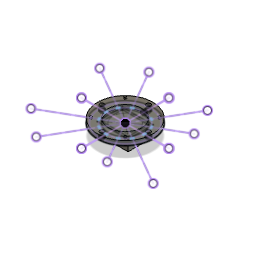
bottom_frame v1 (Autodesk Fusion 360 design; units mm, degrees)
Autodesk Fusion 360 part; units mm, degrees
note: some values were not read from the file. Set by a fixed rule: which sketch regions a step uses.
sketch "스케치1" plane through (0, 0, 0) normal (0, 1, 0) x (1, 0, 0)
  circle A0 centre (0, 0) radius 28 construction
  circle A1 centre (0, 0) radius 38
  circle A2 centre (0, 0) radius 63
  circle A3 centre (0, 0) radius 43 construction
  line L0 (-100, 0) -> (100, 0) construction
  line L1 (0, 100) -> (0, -100) construction
  line L2 (-136.6025, -78.8675) -> (100, 57.735) construction
  line L3 (-137.8994, 79.6163) -> (151.432, -87.4293) construction
  line L4 (-74.5024, -129.042) -> (68.9117, 119.3585) construction
  line L5 (-74.0212, 128.2085) -> (56.0866, -97.1449) construction
  circle A4 centre (0, 0) radius 58 construction
  dimension "d1" = 56
  dimension "d2" = 10
  dimension "d3" = 25
  dimension "d5" = 5
  dimension "d8" = 30
  dimension "d10" = 30
  dimension "d11" = 60
  dimension "d12" = 60
  dimension "d39" = 5
  constraint coincident A0.centre A1.centre
  constraint concentric A0 A1
  constraint concentric A2 A3
  constraint horizontal L0
  constraint vertical L1
  constraint coincident A0.centre L2
  constraint coincident A0.centre L3
  constraint coincident A0.centre L4
  constraint coincident A0.centre L5
  constraint concentric A2 A4
  measures "d1" diameter of A0
  measures "d2" distance of A0 A1
  measures "d3" distance of A1 A2
  measures "d5" distance of A1 A3
  measures "d8" angle of L0 L2
  measures "d10" angle of L0 L3
  measures "d11" angle of L0 L4
  measures "d12" angle of L0 L5
  measures "d39" distance of A2 A4
sketch "스케치2" plane through (0, 0, 0) normal (0, 1, 0) x (1, 0, 0)
  line L0 (-2.5, 45) -> (2.5, 45)
  line L1 (2.5, 45) -> (2.5, 43)
  line L2 (2.5, 43) -> (-2.5, 43)
  line L3 (-2.5, 43) -> (-2.5, 45)
  line L4 (-2.5, 43) -> (2.5, 45) construction
  line L5 (2.5, 43) -> (-2.5, 45) construction
  line L6 (0, 43) -> (0, 45) construction
  line L7 (-43, -2.5) -> (-45, -2.5)
  line L8 (-45, -2.5) -> (-43, 2.5) construction
  line L9 (-43, 2.5) -> (-43, -2.5)
  line L10 (-45, 0) -> (-43, 0) construction
  line L11 (-45, -2.5) -> (-45, 2.5)
  line L12 (-45, 2.5) -> (-43, -2.5) construction
  line L13 (-45, 2.5) -> (-43, 2.5)
  circle A0 centre (0, 0) radius 43
  line L14 (-20.3349, 40.2211) -> (-19.3349, 38.4891)
  line L15 (-24.6651, 37.7211) -> (-20.3349, 40.2211)
  line L16 (-19.3349, 38.4891) -> (-23.6651, 35.9891)
  line L17 (-23.6651, 35.9891) -> (-20.3349, 40.2211) construction
  line L18 (-23.6651, 35.9891) -> (-24.6651, 37.7211)
  line L19 (-19.3349, 38.4891) -> (-24.6651, 37.7211) construction
  line L20 (-21.5, 37.2391) -> (-22.5, 38.9711) construction
  line L21 (-74.0212, 128.2085) -> (56.0866, -97.1449)
  line L22 (-40.2211, 20.3349) -> (-37.7211, 24.6651)
  line L23 (-38.4891, 19.3349) -> (-37.7211, 24.6651) construction
  line L24 (-35.9891, 23.6651) -> (-40.2211, 20.3349) construction
  line L25 (-38.4891, 19.3349) -> (-40.2211, 20.3349)
  line L26 (-37.7211, 24.6651) -> (-35.9891, 23.6651)
  line L27 (-35.9891, 23.6651) -> (-38.4891, 19.3349)
  line L28 (-37.2391, 21.5) -> (-38.9711, 22.5) construction
  line L29 (-137.8994, 79.6163) -> (151.432, -87.4293)
  line L30 (-100, 0) -> (100, 0)
  line L31 (-40.2211, -20.3349) -> (-35.9891, -23.6651) construction
  line L32 (-38.9711, -22.5) -> (-37.2391, -21.5) construction
  line L33 (-35.9891, -23.6651) -> (-37.7211, -24.6651)
  line L34 (-40.2211, -20.3349) -> (-38.4891, -19.3349)
  line L35 (-37.7211, -24.6651) -> (-38.4891, -19.3349) construction
  line L36 (-37.7211, -24.6651) -> (-40.2211, -20.3349)
  line L37 (-38.4891, -19.3349) -> (-35.9891, -23.6651)
  line L38 (-24.6651, -37.7211) -> (-19.3349, -38.4891) construction
  line L39 (-22.5, -38.9711) -> (-21.5, -37.2391) construction
  line L40 (-19.3349, -38.4891) -> (-20.3349, -40.2211)
  line L41 (-24.6651, -37.7211) -> (-23.6651, -35.9891)
  line L42 (-20.3349, -40.2211) -> (-23.6651, -35.9891) construction
  line L43 (-20.3349, -40.2211) -> (-24.6651, -37.7211)
  line L44 (-23.6651, -35.9891) -> (-19.3349, -38.4891)
  line L45 (0, -45) -> (0, -43) construction
  line L46 (2.5, -43) -> (2.5, -45)
  line L47 (2.5, -45) -> (-2.5, -43) construction
  line L48 (-2.5, -45) -> (2.5, -43) construction
  line L49 (-2.5, -43) -> (2.5, -43)
  line L50 (-2.5, -45) -> (-2.5, -43)
  line L51 (2.5, -45) -> (-2.5, -45)
  line L52 (22.5, -38.9711) -> (21.5, -37.2391) construction
  line L53 (23.6651, -35.9891) -> (24.6651, -37.7211)
  line L54 (24.6651, -37.7211) -> (19.3349, -38.4891) construction
  line L55 (20.3349, -40.2211) -> (23.6651, -35.9891) construction
  line L56 (19.3349, -38.4891) -> (23.6651, -35.9891)
  line L57 (20.3349, -40.2211) -> (19.3349, -38.4891)
  line L58 (24.6651, -37.7211) -> (20.3349, -40.2211)
  line L59 (38.9711, -22.5) -> (37.2391, -21.5) construction
  line L60 (38.4891, -19.3349) -> (40.2211, -20.3349)
  line L61 (40.2211, -20.3349) -> (35.9891, -23.6651) construction
  line L62 (37.7211, -24.6651) -> (38.4891, -19.3349) construction
  line L63 (35.9891, -23.6651) -> (38.4891, -19.3349)
  line L64 (37.7211, -24.6651) -> (35.9891, -23.6651)
  line L65 (40.2211, -20.3349) -> (37.7211, -24.6651)
  line L66 (43, 0) -> (45, 0) construction
  line L67 (45, -2.5) -> (43, -2.5)
  line L68 (43, -2.5) -> (45, 2.5) construction
  line L69 (43, 2.5) -> (45, -2.5) construction
  line L70 (45, 2.5) -> (45, -2.5)
  line L71 (43, 2.5) -> (45, 2.5)
  line L72 (43, -2.5) -> (43, 2.5)
  line L73 (37.2391, 21.5) -> (38.9711, 22.5) construction
  line L74 (40.2211, 20.3349) -> (38.4891, 19.3349)
  line L75 (38.4891, 19.3349) -> (37.7211, 24.6651) construction
  line L76 (35.9891, 23.6651) -> (40.2211, 20.3349) construction
  line L77 (37.7211, 24.6651) -> (40.2211, 20.3349)
  line L78 (35.9891, 23.6651) -> (37.7211, 24.6651)
  line L79 (38.4891, 19.3349) -> (35.9891, 23.6651)
  line L80 (21.5, 37.2391) -> (22.5, 38.9711) construction
  line L81 (24.6651, 37.7211) -> (23.6651, 35.9891)
  line L82 (23.6651, 35.9891) -> (20.3349, 40.2211) construction
  line L83 (19.3349, 38.4891) -> (24.6651, 37.7211) construction
  line L84 (20.3349, 40.2211) -> (24.6651, 37.7211)
  line L85 (19.3349, 38.4891) -> (20.3349, 40.2211)
  line L86 (23.6651, 35.9891) -> (19.3349, 38.4891)
  line L87 (-136.6025, -78.8675) -> (100, 57.735)
  line L88 (-74.5024, -129.042) -> (68.9117, 119.3585)
  line L89 (0, 100) -> (0, -100)
  dimension "d13" = 5
  dimension "d14" = 2
  constraint horizontal L0
  constraint vertical L1
  constraint horizontal L2
  constraint vertical L3
  constraint midpoint L2 L6.start
  constraint midpoint L0 L6.end
  constraint midpoint L10.start L11
  constraint midpoint L10.end L9
  constraint tangent L2 A0
  constraint coincident L6.start A0
  constraint midpoint L20.start L16
  constraint midpoint L20.end L15
  constraint perpendicular L16 L18
  constraint perpendicular L14 L16
  constraint perpendicular L14 L15
  constraint collinear L20 L21
  constraint tangent A0 L16
  constraint perpendicular L11 L13
  constraint perpendicular L7 L11
  constraint perpendicular L7 L9
  constraint midpoint L28.start L27
  constraint midpoint L28.end L22
  constraint perpendicular L25 L27
  constraint perpendicular L26 L27
  constraint perpendicular L22 L26
  constraint collinear L28 L29
  constraint tangent A0 L27
  constraint collinear L10 L30
  constraint tangent L9 A0
  constraint midpoint L32.start L36
  constraint midpoint L32.end L37
  constraint perpendicular L34 L36
  constraint perpendicular L33 L36
  constraint perpendicular L33 L37
  constraint midpoint L39.start L43
  constraint midpoint L39.end L44
  constraint perpendicular L41 L43
  constraint perpendicular L40 L43
  constraint perpendicular L40 L44
  constraint midpoint L45.start L51
  constraint midpoint L45.end L49
  constraint perpendicular L50 L51
  constraint perpendicular L46 L51
  constraint perpendicular L46 L49
  constraint midpoint L52.start L58
  constraint midpoint L52.end L56
  constraint perpendicular L57 L58
  constraint perpendicular L53 L58
  constraint perpendicular L53 L56
  constraint midpoint L59.start L65
  constraint midpoint L59.end L63
  constraint perpendicular L64 L65
  constraint perpendicular L60 L65
  constraint perpendicular L60 L63
  constraint midpoint L66.start L72
  constraint midpoint L66.end L70
  constraint perpendicular L71 L72
  constraint perpendicular L67 L72
  constraint perpendicular L67 L70
  constraint midpoint L73.start L79
  constraint midpoint L73.end L77
  constraint perpendicular L78 L79
  constraint perpendicular L74 L79
  constraint perpendicular L74 L77
  constraint midpoint L80.start L86
  constraint midpoint L80.end L84
  constraint perpendicular L85 L86
  constraint perpendicular L81 L86
  constraint perpendicular L81 L84
  constraint collinear L32 L87
  constraint tangent A0 L37
  constraint collinear L39 L88
  constraint tangent A0 L44
  constraint collinear L45 L89
  constraint tangent A0 L49
  constraint collinear L21 L52
  constraint tangent A0 L56
  constraint collinear L29 L59
  constraint tangent A0 L63
  constraint collinear L30 L66
  constraint tangent A0 L72
  constraint collinear L73 L87
  constraint tangent A0 L79
  constraint collinear L80 L88
  constraint tangent A0 L86
  constraint equal L3 L14
  constraint equal L0 L15
  constraint equal L18 L26
  constraint equal L15 L22
  constraint equal L13 L25
  constraint equal L11 L22
  constraint equal L11 L36
  constraint equal L7 L34
  constraint equal L33 L41
  constraint equal L36 L43
  constraint equal L40 L50
  constraint equal L43 L51
  constraint equal L46 L57
  constraint equal L51 L58
  constraint equal L53 L64
  constraint equal L58 L65
  constraint equal L60 L67
  constraint equal L65 L70
  constraint equal L71 L74
  constraint equal L70 L77
  constraint equal L78 L81
  constraint equal L77 L84
  measures "d13" distance of L0.start L0.end
  measures "d14" distance of L0.start L2.end
sketch "스케치3" plane through (0, 0, 0) normal (0, 1, 0) x (1, 0, 0)
  circle A0 centre (53, 0) radius 5
  circle A1 centre (0, 0) radius 58
  line L0 (-100, 0) -> (100, 0)
  circle A2 centre (0, 53) radius 5
  line L1 (0, 100) -> (0, -100)
  circle A3 centre (-53, 0) radius 5
  circle A4 centre (0, -53) radius 5
  line L2 (-30, 23.5) -> (30, 23.5)
  line L3 (30, 23.5) -> (30, -23.5)
  line L4 (30, -23.5) -> (-30, -23.5)
  line L5 (-30, -23.5) -> (-30, 23.5)
  line L6 (-35, 28.5) -> (35, 28.5)
  line L7 (35, 28.5) -> (35, -28.5)
  line L8 (35, -28.5) -> (-35, -28.5)
  line L9 (-35, -28.5) -> (-35, 28.5)
  line L10 (-30, -23.5) -> (30, 23.5) construction
  line L11 (-30, 23.5) -> (30, -23.5) construction
  dimension "d40" = 10
  dimension "d45" = 5
  dimension "d46" = 5
  dimension "d47" = 5
  dimension "d48" = 5
  dimension "d49" = 47
  dimension "d50" = 60
  constraint tangent A0 A1
  constraint coincident A0.centre L0
  constraint tangent A1 A2
  constraint coincident A2.centre L1
  constraint tangent A1 A3
  constraint coincident L0 A3.centre
  constraint tangent A1 A4
  constraint coincident L1 A4.centre
  constraint equal A0 A2
  constraint equal A2 A3
  constraint equal A3 A4
  constraint horizontal L2
  constraint vertical L3
  constraint horizontal L4
  constraint vertical L5
  constraint horizontal L6
  constraint vertical L7
  constraint horizontal L8
  constraint vertical L9
  constraint midpoint L10 A1.centre
  constraint coincident A1.centre origin
  measures "d40" diameter of A0
  measures "d45" distance of L2 L6
  measures "d46" distance of L3 L7
  measures "d47" distance of L5 L9
  measures "d48" distance of L4 L8
  measures "d49" distance of L2.end L3.end
  measures "d50" distance of L3 L5
extrude "돌출1" add sketch "스케치1" along normal blind 10
extrude "돌출2" cut sketch "스케치3" along normal blind 10 contours A0 L0 | A0 L0 | A2 L1 | A2 L1 | L1 A4 | L1 A4 | L0 A3 | L0 A3
extrude "돌출3" add sketch "스케치3" along normal blind 3 contours A0 L0 | A0 L0 | A2 L1 | A2 L1 | L1 A4 | L1 A4 | L0 A3 | L0 A3
extrude "돌출4" add sketch "스케치1" along normal blind 3 contours A1
extrude "돌출5" add sketch "스케치3" against normal blind 20 contours L0 L1 L3 L4 L7 L8 | L0 L1 L2 L3 L6 L7 | L0 L1 L2 L5 L6 L9 | L0 L1 L4 L5 L8 L9
extrude "돌출6" add sketch "스케치3" along normal blind 2 contours A0 L0 | A0 L0 | A2 L1 | A2 L1 | L1 A4 | L1 A4 | L0 A3 | L0 A3
ref_plane "작업 평면1" through (0, 10, 0) normal (0, 1, 0) x (1, 0, 0)
sketch "스케치4" plane through (0, 10, 0) normal (0, 1, 0) x (1, 0, 0)
  line L0 (-66.5161, 66.5161) -> (73.3003, -73.3003) construction
  line L1 (0, 95) -> (0, -90) construction
  line L2 (74.0412, 0) -> (-90, 0) construction
  line L3 (68.1407, 68.1407) -> (-64.9256, -64.9256) construction
  circle A0 centre (0, 0) radius 58 construction
  circle A1 through (58, 0, -10) (-29, 50.2295, -10) (-29, -50.2295, -10)
  circle A2 centre (39.2444, -39.2444) radius 2.5
  circle A3 centre (39.2444, 39.2444) radius 2.5
  circle A4 centre (-39.2444, 39.2444) radius 2.5
  circle A5 centre (-39.2444, -39.2444) radius 2.5
  dimension "d64" = 45
  dimension "d65" = 5
  constraint coincident A0.centre L0
  constraint perpendicular L1 L2
  constraint coincident A0.centre L1
  constraint coincident A0.centre L2
  constraint perpendicular L0 L3
  constraint coincident A0.centre L3
  constraint coincident A0.centre origin
  constraint coincident L0 A2.centre
  constraint tangent A0 A2
  constraint coincident L3 A3.centre
  constraint equal A2 A3
  constraint tangent A0 A3
  constraint coincident L0 A4.centre
  constraint equal A3 A4
  constraint tangent A0 A4
  constraint coincident L3 A5.centre
  constraint tangent A0 A5
  constraint equal A2 A5
  measures "d64" angle of L0 L1
  measures "d65" diameter of A2
extrude "돌출7" add sketch "스케치4" along normal blind 4
extrude "돌출8" cut 4 faces at (39.9052, 14, -39.5924) (-38.5836, 14, -39.5924) (-38.5836, 14, 38.8964) (39.9052, 14, 38.8964) along direction (0, -1, 0) blind 1
extrude "돌출9" add 1 faces at (-10, -20, -26.8333) along direction (0, -1, 0) blind 5
